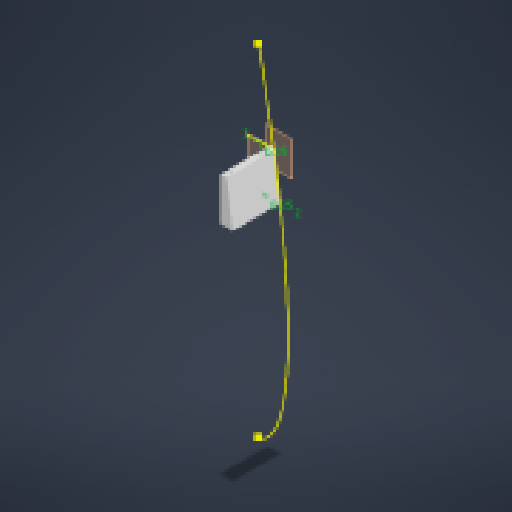
# Autodesk Inventor part: servo cap
Saved by Autodesk Inventor 2026.1 (Build 301233000, 233)
## iProperties
Created: 2025-11-12
Part Number: servo cap
Material: Generic
Document SubType Name: Modeling
Designer: mateo
Density: 1 g/cm^3
Appearance: Default
Author: mateo
Autodesk Inventor part; units mm, degrees
ref_plane "YZ Plane" through (0, 0, 0) normal (1, 0, 0) x (0, 1, 0)
ref_plane "Work Plane1" through (0, 0, 0) normal (0, 0, 1) x (1, 0, 0)
sketch "Sketch1" plane through (0, 0, 0) normal (0, 0, 1) x (1, 0, 0)
  spline S0 degree 3 poles (0.756, 49.6264) (0.8045, 49.3961) (1.4299, 46.4448) (3.02, 38.5419) (3.7417, 34.8308) (6.1255, 22.1808) (7.7131, 13.0519) (12.377, -15.9979) (15.3565, -38.2776) (18.0982, -72.579) (18.7462, -87.3982) (17.8341, -109.2065) (16.9191, -121.3453) (13.1344, -135.1445) (11.7229, -139.4741) (8.6906, -144.8131) (7.5566, -146.4347) (5.361, -148.5489) (4.4031, -149.2519) (2.172, -150.2514) (1.1579, -150.3736) (0.378, -150.3736) knots -21.570573 -21.570573 -21.570573 -21.570573 -20.133907 -20.133907 -18.864962 -18.864962 -15.766925 -15.766925 -8.908038 -8.908038 -4.28709 -4.28709 -1.655649 -1.655649 -0.852769 -0.852769 -0.490947 -0.490947 -0.258162 -0.258162 0 0 0 0 projected
  line L0 (13.2039, -25.771) -> (-6.8, -25.771) projected
  line L1 (-6.8, 0) -> (9.8005, 0) projected
  line L2 (5.2, -2.2181) -> (5.2, 1.2819) projected
  line L3 (6.2, 0) -> (6.2, -25.771)
  line L4 (6.2, -0.25) -> (9.8396, -0.25)
  line L5 (6.2, -25.521) -> (13.4551, -25.521)
  circle A0 centre (8.0198, -0.25) radius 1
  circle A1 centre (8.0783, -25.521) radius 1
  circle A2 centre (8.0198, -0.25) radius 1
  circle A3 centre (8.0783, -25.521) radius 1
  point P0 (0, 0)
  point P1 (9.0783, -25.521)
  point P2 (9.0198, -0.25)
  point P3 (7.0198, -0.25)
  point P4 (7.0783, -25.521)
  dimension "d0" = 1
  dimension "d1" = 0.25
  dimension "d2" = 0.25
  dimension "d3" = 2
  dimension "d4" = 2
  constraints: 6 end point, 5 point on line, 4 centre point, 2 coincident, 2 concentric, 1 horizontal, 1 midpoint, 1 parallel, 1 perpendicular, 2 other
  measures "d0" distance between parallel lines of L3 L2
  measures "d1" distance between parallel lines of L5 L0
  measures "d2" distance between parallel lines of L1 L4
  measures "d3" diameter of A0
  measures "d4" diameter of A1
ref_plane "Work Plane2" through (-6.6501, -24.5518, 27.7072) normal (0, -0.0032, 1) x (1, 0, 0)
ref_plane "Work Plane3" through (-6.6501, -24.5518, 27.7072) normal (0, -0.0032, 1) x (1, 0, 0)
extrude "Extrusion1" add sketch "Sketch1" along normal up to surface contours S0 L5 A1 L3 L4 A0 | A0 L4 | L5 A1 surface through (-6.6501, -24.5518, 27.7072) normal (0, -0.0032, 1)
ref_plane "Work Plane4" through (0, 0, 80) normal (0, 0, 1) x (1, 0, 0)
sketch "Sketch3" plane through (6.2, -0.25, 0) normal (0, 1, 0) x (1, 0, 0)
  circle A0 centre (1.8198, -5) radius 1
  circle A1 centre (1.8198, -17.7838) radius 1
  line L0 (0, -27.7838) -> (3.6396, -27.7838) projected
  line L1 (3.6396, 0) -> (0, 0) projected
  point P0 (-6.2, 0)
  point P1 (1.8198, -27.7838)
  point P2 (1.8198, 0)
  dimension "d10" = 2
  dimension "d11" = 2
  dimension "d13" = 10
  dimension "d14" = 5
  constraints: 2 centre point, 2 midpoint
  measures "d10" diameter of A0
  measures "d11" diameter of A1
  measures "d13" distance of point (1.82, -27.784) A1.centre
  measures "d14" distance of point (1.82, 0) A0.centre
extrude "Extrusion3" add sketch "Sketch3" along normal blind 1
fillet "Fillet1" radius 1 2 edges at (7.0198, 0.75, 5) (7.0198, 0.75, 17.7838)
ref_plane "Work Plane5" through (6.2, -12.8855, 0) normal (0, 1, 0) x (1, 0, 0)
mirror "Mirror2" about plane through (6.2, -12.8855, 0) normal (0, 1, 0) of "Extrusion3"
fillet "Fillet2" radius 1 2 edges at (7.0198, -26.521, 17.7838) (7.0198, -26.521, 5)
ref_plane "Work Plane6" through (0, 0, 792.194) normal (0, 0, 1) x (1, 0, 0)
mirror "Mirror3" about plane through (0, 0, 80) normal (0, 0, 1)
body "Solid1"
